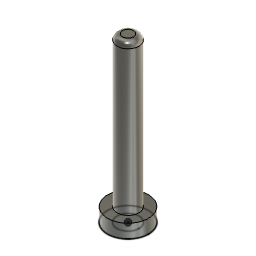
bending_tool_axis v2 (Autodesk Fusion 360 design; units mm, degrees)
Autodesk Fusion 360 part; units mm, degrees
sketch "Skizze1" plane through (0, 0, 0) normal (0, 0, 1) x (1, 0, 0)
  circle A0 centre (0, 0) radius 7.5
  circle A1 centre (0, 0) radius 4
  dimension "d1" = 15
  dimension "d2" = 8
  constraint coincident A0.centre A1.centre
  measures "d1" diameter of A0
  measures "d2" diameter of A1
extrude "Extrusion1" add sketch "Skizze1" along normal blind 5
extrude "Extrusion2" add sketch "Skizze1" along normal blind 60 contours A1
fillet "Abrundung1" radius 2 1 edges at (-3.7293, -1.4465, 60)
